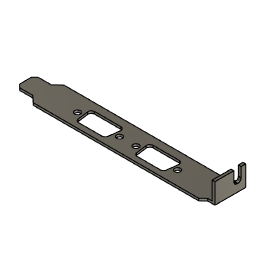
ISA_QuadUART2_bracket (Autodesk Fusion 360 design; units mm, degrees)
Autodesk Fusion 360 part; units mm, degrees
sketch "스케치1" plane through (0, 0, 0) normal (0, 0, 1) x (1, 0, 0)
  line L0 (14, 18.6) -> (114.5, 18.6)
  line L1 (114.5, 18.6) -> (114.5, 0)
  line L2 (114.5, 0) -> (14, 0)
  line L3 (14, 0) -> (14, 18.6)
  line L4 (0, 14.875) -> (10, 14.875)
  line L5 (10, 14.875) -> (10, 3.725)
  line L6 (10, 3.725) -> (0, 3.725)
  line L7 (0, 3.725) -> (0, 14.875)
  line L8 (0, 9.3) -> (10, 9.3) construction
  line L9 (10, 14.875) -> (14, 18.6)
  line L10 (10, 3.725) -> (14, 0)
  line L11 (1.75, 0) -> (22.5, 0)
  line L12 (0, 1.75) -> (0, 22.5)
  line L13 (120, 21.36) -> (117.25, 21.36)
  line L14 (117.25, 21.36) -> (117.25, 2.66)
  line L15 (117.25, 2.66) -> (120, 2.66)
  line L16 (120, 2.66) -> (120, 21.36)
  line L17 (114.5, 0) -> (144, 0) construction
  line L18 (114.5, 18.6) -> (117.25, 21.36)
  line L19 (114.5, 0) -> (117.25, 2.66)
  line L20 (120, 21.36) -> (121.7, 21.36)
  line L21 (121.7, 21.36) -> (121.7, 2.66)
  line L22 (121.7, 2.66) -> (120, 2.66)
  line L23 (120, 2.66) -> (120, 21.36)
  dimension "d1" = 100.5
  dimension "d2" = 18.6
  dimension "d3" = 10
  dimension "d4" = 11.15
  dimension "d5" = 4
  dimension "d6" = 18.7
  dimension "d7" = 2.66
  dimension "d8" = 2.75
  dimension "d9" = 2.75
  dimension "d10" = 1.7
  constraint horizontal L0
  constraint vertical L1
  constraint horizontal L2
  constraint vertical L3
  constraint horizontal L4
  constraint vertical L5
  constraint horizontal L6
  constraint vertical L7
  constraint coincident L7 L8.start
  constraint coincident L5 L8.end
  constraint perpendicular L5 L8
  constraint symmetric L4 L6 L8
  constraint symmetric L0 L2 L8
  constraint collinear L2 L11
  constraint collinear L7 L12
  constraint horizontal L13
  constraint vertical L14
  constraint horizontal L15
  constraint vertical L16
  constraint perpendicular L1 L17
  constraint coincident L0.end L1.start
  constraint coincident L13.end L14.start
  constraint coincident L14.end L15.start
  constraint coincident L1.end L2.start
  constraint horizontal L20
  constraint vertical L21
  constraint horizontal L22
  constraint vertical L23
  measures "d1" distance of L0.start L0.end
  measures "d2" distance of L0.start L2.end
  measures "d3" distance of L4.start L4.end
  measures "d4" distance of L4.start L6.end
  measures "d5" distance of L3 L5
  measures "d6" distance of L13 L15
  measures "d7" distance of L15 L17
  measures "d8" distance of L1 L14
  measures "d9" distance of L14 L16
  measures "d10" distance of L16 L21
extrude "돌출1" add sketch "스케치1" along normal blind 1.4 contours L0 L1 L2 L3 L11 | L3 L5 L9 L10 | L1 L14 L18 L19 | L4 L5 L6 L7 L12 | L13 L14 L15 L16 L23
extrude "돌출2" add sketch "스케치1" along normal blind 12.4 contours L16 L20 L21 L22 L23
chamfer "모따기1" distance 2 angle 45 2 edges at (0, 3.725, 0.7) (0, 14.875, 0.7)
sketch "스케치2" plane through (121.7, 0, 0) normal (1, 0, 0) x (0, 1, 0)
  line L0 (2.66, 0) -> (21.36, 0)
  line L1 (21.36, 0) -> (21.36, 12.4)
  line L2 (21.36, 12.4) -> (2.66, 12.4)
  line L3 (2.66, 12.4) -> (2.66, 0)
  line L4 (14.16, 12.4) -> (18.56, 12.4)
  line L5 (18.56, 12.4) -> (18.56, 4.5)
  line L6 (18.56, 4.5) -> (14.16, 4.5)
  line L7 (14.16, 4.5) -> (14.16, 12.4)
  dimension "d16" = 2.8
  dimension "d17" = 4.4
  dimension "d18" = 7.9
  constraint horizontal L4
  constraint vertical L5
  constraint horizontal L6
  constraint vertical L7
  constraint collinear L2 L4
  measures "d16" distance of L1 L5
  measures "d17" distance of L5.end L6.end
  measures "d18" distance of L4.end L5.end
extrude "돌출3" cut sketch "스케치2" against normal blind 3 contours L2 L4 L5 L6 L7
fillet "모깎기1" radius 2 2 edges at (120.85, 14.16, 4.5) (120.85, 18.56, 4.5)
sketch "스케치3" plane through (0, 0, 1.4) normal (0, 0, 1) x (-1, 0, 0)
  line L0 (-2, -14.875) -> (0, -12.875)
  line L1 (0, -12.875) -> (0, -5.725)
  line L2 (0, -5.725) -> (-2, -3.725)
  line L3 (-2, -3.725) -> (-10, -3.725)
  line L4 (-10, -3.725) -> (-14, 0)
  line L5 (-14, 0) -> (-114.5, 0)
  line L6 (-114.5, 0) -> (-117.25, -2.66)
  line L7 (-117.25, -2.66) -> (-120, -2.66)
  line L8 (-120, -2.66) -> (-120, -21.36)
  line L9 (-120, -21.36) -> (-117.25, -21.36)
  line L10 (-117.25, -21.36) -> (-114.5, -18.6)
  line L11 (-114.5, -18.6) -> (-14, -18.6)
  line L12 (-14, -18.6) -> (-10, -14.875)
  line L13 (-10, -14.875) -> (-2, -14.875)
  line L14 (7.5, -3.3) -> (-137.5, -3.3) construction
  line L15 (-114.5, 0) -> (-14, 0)
  line L16 (7.5, -14) -> (-137.5, -14) construction
  line L17 (-70.5, -14) -> (-91, -14)
  line L18 (-71.9, -3.3) -> (-89.6, -3.3)
  line L19 (-70.5, -14) -> (-71.9, -3.3)
  line L20 (-91, -14) -> (-89.6, -3.3)
  line L21 (-80.75, -32) -> (-80.75, 14) construction
  line L22 (-70.5, -26) -> (-70.5, 12) construction
  line L23 (-91, -26) -> (-91, 12) construction
  circle A0 centre (-67.995, -8.4) radius 1.8
  circle A1 centre (-93.205, -8.4) radius 1.8
  line L24 (-91.405, -12) -> (-91.405, -5.5195) construction
  line L25 (-69.795, -12) -> (-69.795, -5.5195) construction
  line L26 (-66.5, -6.6) -> (-95, -6.6) construction
  line L27 (-35, -14) -> (-55.5, -14)
  line L28 (-36.4, -3.3) -> (-54.1, -3.3)
  line L29 (-35, -14) -> (-36.4, -3.3)
  line L30 (-55.5, -14) -> (-54.1, -3.3)
  circle A2 centre (-32.495, -8.4) radius 1.8
  circle A3 centre (-58.005, -8.4) radius 1.8
  line L31 (-35, -26) -> (-35, 12) construction
  line L32 (-55.5, -26) -> (-55.5, 12) construction
  line L33 (-34.295, -12) -> (-34.295, -5.5195) construction
  line L34 (-56.205, -12) -> (-56.205, -5.5195) construction
  dimension "d23" = 3.3
  dimension "d24" = 10.7
  dimension "d25" = 20.5
  dimension "d26" = 17.7
  dimension "d27" = 29
  dimension "d28" = 3.6
  dimension "d30" = 0.705
  dimension "d31" = 0.405
  dimension "d32" = 3.3
  dimension "d37" = 3.6
  dimension "d38" = 0.705
  dimension "d39" = 0.705
  dimension "d40" = 15
  constraint perpendicular L8 L14
  constraint parallel L16 L17
  constraint parallel L11 L18
  constraint perpendicular L15 L21
  constraint symmetric L17.start L17.end L21
  constraint symmetric L18.start L18.end L21
  constraint collinear L14 L18
  constraint collinear L16 L17
  constraint vertical L22
  constraint vertical L23
  constraint coincident L17.end L23
  constraint coincident L17.start L22
  constraint equal A0 A1
  constraint perpendicular L16 L24
  constraint tangent A1 L24
  constraint tangent A0 L25
  constraint perpendicular L24 L26
  constraint symmetric L21 L26.start L26.end
  constraint tangent A1 L26
  constraint tangent A0 L26
  constraint parallel L16 L27
  constraint parallel L16 L28
  constraint equal L17 L27
  constraint equal L18 L28
  constraint equal L20 L30
  constraint equal L19 L29
  constraint collinear L16 L27
  constraint equal A2 A3
  constraint vertical L31
  constraint vertical L32
  constraint coincident L27.start L31
  constraint coincident L27.end L32
  constraint tangent A2 L33
  constraint tangent A3 L34
  measures "d23" distance of L14 L15
  measures "d24" distance of L14 L16
  measures "d25" distance of L17.start L17.end
  measures "d26" distance of L18.start L18.end
  measures "d27" distance of L8 L23
  measures "d28" diameter of A0
  measures "d30" distance of L22 L25
  measures "d31" distance of L23 L24
  measures "d32" distance of L14 L26
  measures "d37" diameter of A2
  measures "d38" distance of L32 L34
  measures "d39" distance of L31 L33
  measures "d40" distance of L22 L32
extrude "돌출4" cut sketch "스케치3" against normal blind 2 contours L17 L18 L19 L20 | A0 | A1
fillet "모깎기2" radius 2 4 edges at (91, 14, 0.7) (70.5, 14, 0.7) (89.6, 3.3, 0.7) (71.9, 3.3, 0.7)
extrude "돌출5" cut sketch "스케치3" against normal blind 4 contours L27 L28 L29 L30 | A2 | A3
fillet "모깎기3" radius 2 4 edges at (35, 14, 0.7) (55.5, 14, 0.7) (36.4, 3.3, 0.7) (54.1, 3.3, 0.7)
named bodies: "body 1"
